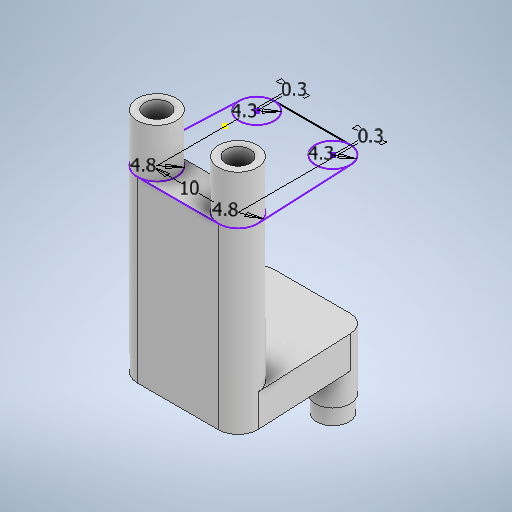
# Autodesk Inventor part: gripper3rightsideservoholder
Saved by Autodesk Inventor 2025.2 (Build 292293000, 293)
## iProperties
Created: 2025-03-30
Part Number: gripper3rightsideservoholder
Material: Generic
Document SubType Name: Modeling
Designer: m_kni
Density: 1 g/cm^3
Appearance: Default
Author: m_kni
## iProperties of the stored document gripper3rightsideservoholder_3DPrint.ipt
Created: 2025-04-02
Part Number: gripper3rightsideservoholder_3DPrint
Material: Generic
Document SubType Name: Modeling
Designer: m_kni
Density: 1 g/cm^3
Appearance: Default
Author: m_kni
Autodesk Inventor part; units mm, degrees
ref_plane "YZ Plane" through (0, 0, 0) normal (1, 0, 0) x (0, 1, 0)
ref_plane "XZ Plane" through (0, 0, 0) normal (0, 1, 0) x (-1, 0, 0)
ref_plane "XY Plane" through (0, 0, 0) normal (0, 0, 1) x (1, 0, 0)
sketch "Sketch1" plane through (0, 0, 0) normal (0, 1, 0) x (-1, 0, 0)
  circle A0 centre (-0.062958, 8.481909) radius 2.4
  circle A1 centre (-0.362958, -3.518091) radius 2.15
  circle A2 centre (-10.062958, 8.481909) radius 2.4
  circle A3 centre (-9.762958, -3.518091) radius 2.15
  point P0 (0, 0)
  dimension "d0" = 4.8
  dimension "d1" = 4.3
  dimension "d3" = 4.8
  dimension "d5" = 4.3
  dimension "d24" = 10
  dimension "d25" = 0.3
  dimension "d26" = 0.3
  constraints: 4 centre point, 1 coincident
  measures "d0" diameter of A0
  measures "d1" diameter of A1
  measures "d3" diameter of A2
  measures "d5" diameter of A3
  measures "d24" distance of point (-0.063, 8.482) A2.centre
  measures "d25" horizontal distance of A3.centre A2.centre
  measures "d26" horizontal distance of point (-0.063, 8.482) A1.centre
extrude "Extrusion1" add sketch "Sketch1" along normal blind 6 contours A0 | A2
sketch "Sketch2" plane through (0.062958, 0, 8.481909) normal (0, -1, 0) x (1, 0, 0)
  circle A0 centre (0.3, -12) radius 2.15
  circle A1 centre (9.7, -12) radius 2.15
  circle A2 centre (10, 0) radius 2.4
  circle A3 centre (0, 0) radius 2.4
  line L0 (-2.4, 0) -> (-1.85, -12)
  line L1 (0.3, -14.15) -> (9.7, -14.15)
  line L2 (11.85, -12) -> (12.39746, -0.110392)
  line L3 (0, 2.4) -> (10, 2.4)
  point P0 (-0.062958, -8.481909)
  constraints: 8 end point, 8 point on circle, 2 horizontal, 2 tangent
sketch "Sketch3" plane through (0.062958, 0, 8.481909) normal (0, -1, 0) x (1, 0, 0)
  circle A0 centre (10, 0) radius 2.4
  circle A1 centre (0, 0) radius 2.4
  line L0 (0, -2.4) -> (10, -2.4)
  line L1 (0, -2.4) -> (10, -2.4)
  circle A2 centre (0, 0) radius 2.4
  circle A3 centre (10, 0) radius 2.4
  circle A4 centre (10, 0) radius 2.4
  circle A5 centre (0, 0) radius 2.4
  circle A6 centre (0, 0) radius 2.4
  circle A7 centre (0, 0) radius 2.4
  circle A8 centre (0, 0) radius 2.4
  circle A9 centre (10, 0) radius 2.4
  circle A10 centre (10, 0) radius 2.4
  circle A11 centre (10, 0) radius 2.4
  circle A12 centre (10, 0) radius 2.4
  circle A13 centre (0, 0) radius 2.4
  circle A14 centre (10, 0) radius 2.4
  circle A15 centre (10, 0) radius 2.4
  circle A16 centre (0, 0) radius 2.4
  line L2 (0, 2.4) -> (10, 2.4)
  point P0 (-0.062958, -8.481909)
  point P1 (-2.4, 0)
  point P2 (12.39746, -0.110392)
extrude "Extrusion2" add sketch "Sketch3" along normal blind 18
sketch "Sketch4" plane through (0.062958, -18, 8.481909) normal (0, -1, 0) x (1, 0, 0)
  circle A0 centre (0.3, -12) radius 2.15
  circle A1 centre (9.7, -12) radius 2.15
  circle A2 centre (0, 0) radius 2.4
  circle A3 centre (10, 0) radius 2.4
  arc A4 (0, -2.4) -> (0, 2.4) centre (0, 0) ccw
  arc A5 (10, 2.4) -> (10, -2.4) centre (10, 0) ccw
  arc A6 (0, 2.4) -> (0, -2.4) centre (0, 0) ccw
  arc A7 (10, -2.4) -> (10, 2.4) centre (10, 0) ccw
  line L0 (0, -2.4) -> (10, -2.4)
  line L1 (0, -2.4) -> (10, -2.4)
  line L2 (10, 2.4) -> (0, 2.4)
  line L3 (10, 2.4) -> (0, 2.4)
  circle A8 centre (0, 0) radius 2.4
  arc A9 (0, -2.4) -> (0, 2.4) centre (0, 0) ccw
  arc A10 (0, 2.4) -> (0, -2.4) centre (0, 0) ccw
  circle A11 centre (10, 0) radius 2.4
  arc A12 (10, 2.4) -> (10, -2.4) centre (10, 0) ccw
  arc A13 (10, -2.4) -> (10, 2.4) centre (10, 0) ccw
  arc A14 (10, 2.4) -> (10, -2.4) centre (10, 0) ccw
  line L4 (0, -2.4) -> (10, -2.4)
  arc A15 (0, -2.4) -> (0, 2.4) centre (0, 0) ccw
  line L5 (10, 2.4) -> (0, 2.4)
  line L6 (0, -2.4) -> (10, -2.4)
  arc A16 (10, -2.4) -> (10, 2.4) centre (10, 0) ccw
  line L7 (10, 2.4) -> (0, 2.4)
  arc A17 (0, 2.4) -> (0, -2.4) centre (0, 0) ccw
  line L8 (0, -2.4) -> (10, -2.4)
  line L9 (0, -2.4) -> (10, -2.4)
  line L10 (10, 2.4) -> (0, 2.4)
  line L11 (10, 2.4) -> (0, 2.4)
  circle A18 centre (0, 0) radius 2.4
  circle A19 centre (10, 0) radius 2.4
  circle A20 centre (0, 0) radius 2.4
  circle A21 centre (10, 0) radius 2.4
  circle A22 centre (0.3, -12) radius 2.15
  circle A23 centre (9.7, -12) radius 2.15
  circle A24 centre (10, 0) radius 2.4
  circle A25 centre (0, 0) radius 2.4
  line L12 (-2.4, 0) -> (-1.85, -12)
  line L13 (0.3, -14.15) -> (9.7, -14.15)
  line L14 (11.85, -12) -> (12.39746, -0.110392)
  line L15 (0, 2.4) -> (10, 2.4)
  point P0 (-0.062958, -8.481909)
  point P1 (-0.062958, -8.481909)
  point P2 (-0.062958, -8.481909)
  constraints: 5 other
sketch "Sketch4 outline for Extrusion3" plane through (0.062958, -18, 8.481909) normal (0, -1, 0) x (1, 0, 0)
  line L0 (-2.4, 0) -> (-1.85, -12)
  arc A0 (0, 2.4) -> (-2.4, 0) centre (0, 0) ccw
  line L1 (10, 2.4) -> (0, 2.4)
  arc A1 (12.39746, -0.110392) -> (10, 2.4) centre (10, 0) ccw
  line L2 (11.85, -12) -> (12.39746, -0.110392)
  arc A2 (9.7, -14.15) -> (11.85, -12) centre (9.7, -12) ccw
  line L3 (0.3, -14.15) -> (9.7, -14.15)
  arc A3 (-1.85, -12) -> (0.3, -14.15) centre (0.3, -12) ccw
extrude "Extrusion3" add sketch "Sketch4 outline for Extrusion3" along normal blind 4
sketch "Sketch5" plane through (0.062958, -22, 8.481909) normal (0, -1, 0) x (1, 0, 0)
  arc A0 (-1.85, -12) -> (0.3, -14.15) centre (0.3, -12) ccw projected
  circle A1 centre (0.3, -12) radius 2.15
  arc A2 (9.7, -14.15) -> (11.85, -12) centre (9.7, -12) ccw projected
  circle A3 centre (9.7, -12) radius 2.15
  point P0 (-0.062958, -8.481909)
  point P1 (0.3, -14.15)
  constraints: 2 centre point, 2 coincident
extrude "Extrusion4" add sketch "Sketch5" along normal blind 3.5
sketch "Sketch6" plane through (0.362958, -25.5, -3.518091) normal (0, -1, 0) x (1, 0, 0)
  arc A0 (0, -2.15) -> (-2.15, 0) centre (0, 0) ccw projected
  circle A1 centre (0, 0) radius 2
  arc A2 (11.55, 0) -> (9.4, -2.15) centre (9.4, 0) ccw projected
  circle A3 centre (9.4, 0) radius 2
  point P0 (-0.362958, 3.518091)
  dimension "d15" = 4
  dimension "d16" = 4
  constraints: 2 centre point, 2 coincident
  measures "d15" diameter of A1
  measures "d16" diameter of A3
extrude "Extrusion5" add sketch "Sketch6" along normal blind 2
sketch "Sketch7" plane through (0.362958, -27.5, -3.518091) normal (0, -1, 0) x (1, 0, 0)
  circle A0 centre (0, 0) radius 1.5
  circle A1 centre (9.4, 0) radius 2 projected
  circle A2 centre (9.4, 0) radius 1.5
  point P0 (-0.362958, 3.518091)
  dimension "d19" = 3
  dimension "d20" = 3
  constraints: 2 centre point, 1 coincident
  measures "d19" diameter of A0
  measures "d20" diameter of A2
extrude "Extrusion6" cut sketch "Sketch7" against normal blind 6 contours A0 | A2
sketch "Sketch8" plane through (0.062958, 6, 8.481909) normal (0, 1, 0) x (1, 0, 0)
  circle A0 centre (0, 0) radius 1.5
  circle A1 centre (10, 0) radius 2.4 projected
  circle A2 centre (10, 0) radius 1.5
  point P0 (-0.062958, 8.481909)
  dimension "d27" = 3
  dimension "d28" = 3
  constraints: 2 centre point, 1 coincident
  measures "d27" diameter of A0
  measures "d28" diameter of A2
extrude "Extrusion7" cut sketch "Sketch8" against normal blind 10 contours A0 | A2
body "Solid1"
